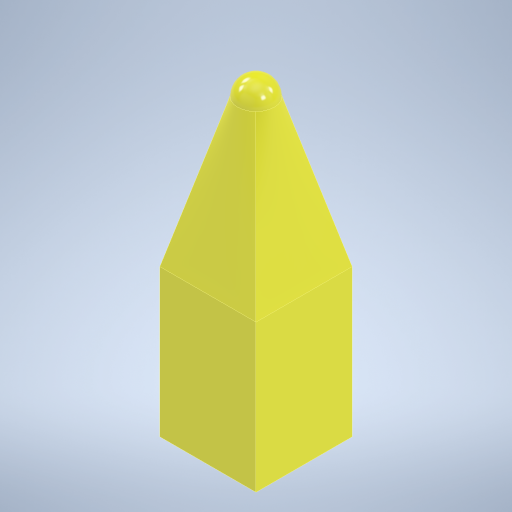
# Autodesk Inventor part: Pies
Saved by Autodesk Inventor 2023 (Build 270158000, 158)
## iProperties
Created: 2024-01-16
Part Number: Pies
Material: PET Plastic
Document SubType Name: Modeling
Designer: juanp
Density: 1.541 g/cm^3
Appearance: Yellow
Author: juanp
Autodesk Inventor part; units mm, degrees
ref_plane "YZ Plane" through (0, 0, 0) normal (1, 0, 0) x (0, 1, 0)
ref_plane "XZ Plane" through (0, 0, 0) normal (0, 1, 0) x (-1, 0, 0)
sketch "Sketch2" plane through (0, 0, 0) normal (0, 1, 0) x (-1, 0, 0)
  line L0 (10.05, 10.05) -> (-10.05, 10.05)
  line L1 (-10.05, 10.05) -> (-10.05, -10.05)
  line L2 (-10.05, -10.05) -> (10.05, -10.05)
  line L3 (10.05, -10.05) -> (10.05, 10.05)
  line L4 (10.05, 10.05) -> (-10.05, -10.05) construction
  line L5 (-10.05, 10.05) -> (10.05, -10.05) construction
  line L6 (13.05, 13.05) -> (-13.05, 13.05)
  line L7 (-13.05, 13.05) -> (-13.05, -13.05)
  line L8 (-13.05, -13.05) -> (13.05, -13.05)
  line L9 (13.05, -13.05) -> (13.05, 13.05)
  point P0 (0, 0)
  dimension "d19" = 20.1
  dimension "d20" = 3
  constraints: 20 end point, 4 parallel, 3 perpendicular, 2 midpoint, 1 horizontal, 3 other
  measures "d19" distance of L2.end L1.end
  measures "d20" distance between parallel lines of L3 L9
extrude "Extrusion2" add sketch "Sketch2" along normal blind 40
ref_plane "Work Plane1" through (0, 80, 0) normal (0, 1, 0) x (1, 0, 0)
sketch "Sketch3" plane through (0, 80, 0) normal (0, 1, 0) x (1, 0, 0)
  line L0 (-10.05, -10.05) -> (-10.05, 10.05) projected
  line L1 (10.05, 10.05) -> (10.05, -10.05) projected
  line L2 (-10.05, -10.05) -> (10.05, 10.05) construction
  circle A0 centre (0, 0) radius 5
  dimension "d24" = 10
  constraints: 2 end point, 1 centre point, 1 coincident
  measures "d24" diameter of A0
sketch "Sketch4" plane through (0, 40, 0) normal (0, 1, 0) x (1, 0, 0)
  line L0 (13.05, -13.05) -> (13.05, 13.05) projected
  line L1 (13.05, 13.05) -> (-13.05, 13.05) projected
  line L2 (-13.05, 13.05) -> (-13.05, -13.05) projected
  line L3 (-13.05, -13.05) -> (13.05, -13.05) projected
  line L4 (-10.05, -10.05) -> (-10.05, 10.05) construction
  line L5 (-10.05, 10.05) -> (10.05, 10.05) projected
  line L6 (10.05, 10.05) -> (10.05, -10.05) projected
  line L7 (10.05, -10.05) -> (-10.05, -10.05) projected
  point P0 (0, 0)
loft "Loft1" add profiles "Sketch3", "Sketch4"
sketch "Sketch5" plane through (0, 80, 0) normal (0, 1, 0) x (1, 0, 0)
  arc A0 (-3.5355, 3.5355) -> (-3.5355, -3.5355) centre (0, 0) ccw projected
  line L0 (-5, 0) -> (5, 0)
  arc A1 (3.5355, -3.5355) -> (3.5355, 3.5355) centre (0, 0) ccw projected
  arc A2 (-3.5355, -3.5355) -> (3.5355, -3.5355) centre (0, 0) ccw projected
  arc A3 (3.5355, -3.5355) -> (3.5355, 3.5355) centre (0, 0) ccw projected
  arc A4 (3.5355, 3.5355) -> (-3.5355, 3.5355) centre (0, 0) ccw projected
  arc A5 (-3.5355, 3.5355) -> (-3.5355, -3.5355) centre (0, 0) ccw projected
  point P0 (-3.5355, -3.5355)
  constraints: 2 end point, 2 point on circle, 1 horizontal, 1 line through centre
revolve "Revolution1" add sketch "Sketch5" angle 360 about axis through (-5, 80, 0) along (1, 0, 0) contours L0 A1 A2 A0
sketch "Sketch6" plane through (-13.05, 0, -13.05) normal (-1, 0, 0) x (0, 0, 1)
  line L0 (9.5145, 80) -> (0, 40) projected
  line L1 (26.1, 0) -> (26.1, 40) projected
  line L2 (0, 40) -> (26.1, 0) construction
  circle A0 centre (13.05, 20) radius 2.15
  point P0 (13.05, 0)
  dimension "d30" = 4.3
  constraints: 2 end point, 1 centre point, 1 midpoint
  measures "d30" diameter of A0
extrude "Extrusion3" cut sketch "Sketch6" against normal blind 18.855
equation "\"l1\" = 1"
body "Solid2"
